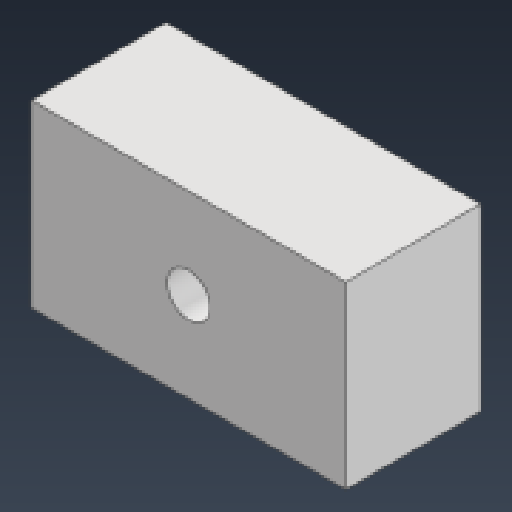
# Autodesk Inventor part: claw_nut_test
Saved by Autodesk Inventor 2023 (Build 270158000, 158)
## iProperties
Created: 2026-01-23
Part Number: claw_nut_test
Material: Generic
Document SubType Name: Modeling
Designer: szymo
Density: 1 g/cm^3
Appearance: Default
Author: szymo
Autodesk Inventor part; units mm, degrees
ref_plane "YZ Plane" through (0, 0, 0) normal (1, 0, 0) x (0, 1, 0)
ref_plane "XZ Plane" through (0, 0, 0) normal (0, 1, 0) x (-1, 0, 0)
ref_plane "XY Plane" through (0, 0, 0) normal (0, 0, 1) x (1, 0, 0)
sketch "Sketch1" plane through (0, 0, 0) normal (0, 0, 1) x (1, 0, 0)
  line L0 (-17.5, 4.45) -> (17.5, 4.45)
  line L1 (17.5, 4.45) -> (17.5, -15.55)
  line L2 (17.5, -15.55) -> (-17.5, -15.55)
  line L3 (-17.5, -15.55) -> (-17.5, 4.45)
  circle A0 centre (0, -5.55) radius 1.8 construction
  line L4 (-17.5, 4.45) -> (17.5, -15.55) construction
  line L5 (17.5, 4.45) -> (-17.5, -15.55) construction
  point P0 (0, 0)
  dimension "d0" = 35
  dimension "d1" = 20
  constraints: 12 end point, 2 parallel, 1 coincident, 1 horizontal, 1 midpoint, 1 perpendicular
  measures "d0" distance of L1.end L2.end
  measures "d1" distance of L0.end L1.end
extrude "Extrusion1" add sketch "Sketch1" against normal blind 15
sketch "Sketch2" plane through (0, 0, -15) normal (0, 0, -1) x (-1, 0, 0)
  circle A0 centre (0, -5.55) radius 2.6 projected
  point P0 (0, 0)
hole "Hole1" at (0, -5.55, -15) direction (0, 0, 1) diameter 4.8 end through all countersink diameter 10 countersink angle 90 clearance for "Countersunk Flat Head Screw ISO 2009/7046" size "M4" standard "ISO"
body "Solid1"
